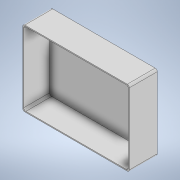
# Autodesk Inventor part: water_bowl
Saved by Autodesk Inventor 2020.3 (Build 243373000, 373)
## iProperties
Created: 2020-12-20
Part Number: water_bowl
Material: 一般
Document SubType Name: Modeling
Designer: touhu_zn72wdq
Density: 1 g/cm^3
Appearance: 既定
Author: touhu_zn72wdq
Autodesk Inventor part; units mm, degrees
ref_plane "YZ Plane" through (0, 0, 0) normal (1, 0, 0) x (0, 1, 0)
ref_plane "XZ Plane" through (0, 0, 0) normal (0, 1, 0) x (-1, 0, 0)
ref_plane "XY Plane" through (0, 0, 0) normal (0, 0, 1) x (1, 0, 0)
sketch "スケッチ1" plane through (0, 0, 0) normal (0, 0, 1) x (1, 0, 0)
  line L0 (75, -52.5) -> (-75, -52.5)
  line L1 (-75, -52.5) -> (-75, 52.5)
  line L2 (-75, 52.5) -> (75, 52.5)
  line L3 (75, 52.5) -> (75, -52.5)
  line L4 (75, -52.5) -> (-75, 52.5) construction
  line L5 (-75, -52.5) -> (75, 52.5) construction
  line L6 (76.5, -54) -> (-76.5, -54)
  line L7 (-76.5, -54) -> (-76.5, 54)
  line L8 (-76.5, 54) -> (76.5, 54)
  line L9 (76.5, 54) -> (76.5, -54)
  line L10 (76.5, -54) -> (-76.5, 54) construction
  line L11 (-76.5, -54) -> (76.5, 54) construction
  point P0 (0, 0)
  dimension "d0" = 150
  dimension "d1" = 105
  dimension "d4" = 153
  dimension "d5" = 108
  constraints: 24 end point, 4 midpoint, 4 parallel, 2 horizontal, 2 perpendicular
  measures "d0" distance of L1.end L2.end
  measures "d1" distance of L0.end L1.end
  measures "d4" distance of L7.end L8.end
  measures "d5" distance of L6.end L7.end
extrude "押し出し1" add sketch "スケッチ1" along normal blind 40
extrude "押し出し2" add sketch "スケッチ1" along normal blind 3 contours L0 L1 L2 L3
fillet "フィレット3" radius 3 4 edges at (-76.5, 54, 20) (-76.5, -54, 20) (76.5, -54, 20) (76.5, 54, 20)
fillet "フィレット3" radius 3 4 edges at (-75, 52.5, 21.5) (75, 52.5, 21.5) (-75, -52.5, 21.5) (75, -52.5, 21.5)
